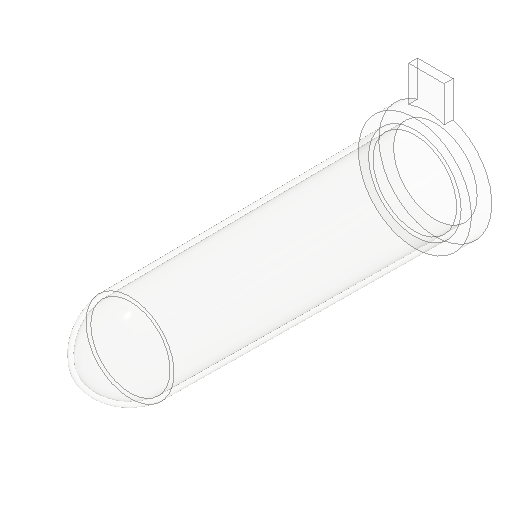
# Autodesk Inventor part: COTS_Eppendorf_10ml_test_tube
Saved by Autodesk Inventor 2026.1 (Build 301233000, 233)
## iProperties
Created: 2017-05-26
Part Number: COTS_Eppendorf_10ml_test_tube
Material: Ogólny
Document SubType Name: Modeling
Designer: Andrzej
Density: 1 g/cm^3
Appearance: Poliwęglan — przezroczysty
Author: Andrzej
Autodesk Inventor part; units mm, degrees
ref_plane "YZ Plane" through (0, 0, 0) normal (1, 0, 0) x (0, 1, 0)
ref_plane "XZ Plane" through (0, 0, 0) normal (0, 1, 0) x (-1, 0, 0)
ref_plane "XY Plane" through (0, 0, 0) normal (0, 0, 1) x (1, 0, 0)
sketch "Szkic1" plane through (0, 0, 0) normal (0, 0, 1) x (1, 0, 0)
  line L0 (0, 13.2758) -> (0, -36.7242)
  line L1 (-5.2, 4.5142) -> (-4.95, -27.4858)
  arc A0 (-4.95, -27.4858) -> (0, -33.4858) centre (2.3877, -26.4741) ccw
  line L2 (-4.7, 4.5142) -> (-4.4503, -27.449)
  arc A1 (-4.4503, -27.449) -> (0, -32.9554) centre (2.3877, -26.4741) ccw
  line L3 (-5.2, 4.5142) -> (-4.7, 4.5142)
  point P0 (0, 0)
  dimension "d0" = 50
  dimension "d1" = 5.2
  dimension "d2" = 4.95
  dimension "d3" = 32
  dimension "d4" = 38
  dimension "d5" = 0.5
  constraints: 8 end point, 4 point on circle, 2 centre point, 2 point on line, 1 horizontal, 1 vertical
  measures "d0" distance of L0.start L0.end
  measures "d1" distance from line of L0 L1.start
  measures "d2" distance from line of L0 L1.end
  measures "d3" vertical distance of L1.end L1.start
  measures "d4" vertical distance of L1.start A0.end
  measures "d5" distance between parallel lines of L1 L2
revolve "Obrót1" add sketch "Szkic1" angle 360 about axis through (0, 13.2758, 0) along (0, -1, 0)
sketch "Szkic2" plane through (0, 4.5142, 0) normal (0, 1, 0) x (1, 0, 0)
  circle A0 centre (0, 0) radius 6.35
  circle A1 centre (0, 0) radius 5.2 projected
  circle A2 centre (0, 0) radius 4.7 projected
  dimension "d7" = 12.7
  constraints: 1 centre point, 1 coincident
  measures "d7" diameter of A0
extrude "Wyciągnięcie proste1" add sketch "Szkic2" along normal blind 2.3 contours A0 | A1
sketch "Szkic3" plane through (0, 6.8142, 0) normal (0, 1, 0) x (1, 0, 0)
  circle A0 centre (0, 0) radius 4.7 projected
  circle A1 centre (0, 0) radius 6.35 projected
  line L0 (2, -10.0268) -> (-2, -10.0268)
  line L1 (2, -10.0268) -> (2, -6.0268)
  line L2 (-2, -10.0268) -> (-2, -6.0268)
  point P0 (0, 0)
  dimension "d10" = 4
  dimension "d11" = 2
  dimension "d12" = 4
  constraints: 6 end point, 2 point on circle, 2 vertical, 1 horizontal
  measures "d10" distance of L0.start L0.end
  measures "d11" horizontal distance of A0.centre L0.end
  measures "d12" distance of L0.start L1.end
extrude "Wyciągnięcie proste2" add sketch "Szkic3" against normal blind 1 contours A1 L1 L0 L2
